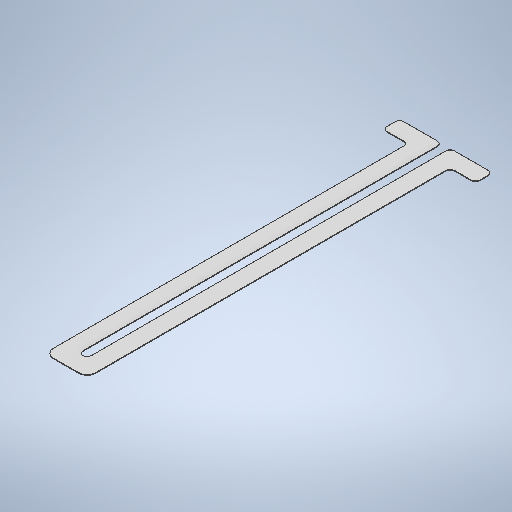
# Autodesk Inventor part: Lungo
Saved by Autodesk Inventor 2025.4 (Build 294407000, 407)
## iProperties
Created: 2026-04-15
Part Number: Lungo
Material: Generic
Document SubType Name: Modeling
Designer: gdira
Density: 1 g/cm^3
Appearance: Default
Author: gdira
Autodesk Inventor part; units mm, degrees
ref_plane "YZ Plane" through (0, 0, 0) normal (1, 0, 0) x (0, 1, 0)
ref_plane "XZ Plane" through (0, 0, 0) normal (0, 1, 0) x (-1, 0, 0)
ref_plane "XY Plane" through (0, 0, 0) normal (0, 0, 1) x (1, 0, 0)
sketch "Sketch1" plane through (0, 0, 0) normal (0, 1, 0) x (-1, 0, 0)
  line L0 (0.1981, -3.9947) -> (-1.7926, -3.9947)
  line L1 (-5.7926, -3.9915) -> (-13.7926, -3.9915)
  line L2 (0.1981, -3.9947) -> (6.2092, -3.9837)
  line L3 (-4.7926, 81.0108) -> (-4.7926, -2.9915)
  line L4 (-2.7926, -2.9947) -> (-2.7926, 81.0108)
  line L5 (-3.7926, 82.0108) -> (-3.7926, 82.0108)
  line L6 (-8.7926, 84.0108) -> (-8.7926, 4.0085)
  line L7 (-6.7926, 86.0108) -> (-0.7926, 86.0108)
  line L8 (1.2074, 84.0108) -> (1.2074, 4.0363)
  arc A0 (-6.7926, 86.0108) -> (-8.7926, 84.0108) centre (-6.7926, 84.0108) ccw
  arc A1 (1.2074, 84.0108) -> (-0.7926, 86.0108) centre (-0.7926, 84.0108) ccw
  line L9 (7.2074, -2.9837) -> (7.2074, -0.9819)
  line L10 (6.2074, 0.0181) -> (2.2074, 0.0181)
  line L11 (1.2074, 1.0181) -> (1.2074, 7.5905)
  line L12 (-14.7926, -2.9915) -> (-14.7926, -0.9915)
  line L13 (-13.7926, 0.0085) -> (-9.7926, 0.0085)
  line L14 (-8.7926, 1.0085) -> (-8.7926, 4.0085)
  arc A2 (-9.7926, 0.0085) -> (-8.7926, 1.0085) centre (-9.7926, 1.0085) ccw
  arc A3 (-13.7926, 0.0085) -> (-14.7926, -0.9915) centre (-13.7926, -0.9915) ccw
  arc A4 (-14.7926, -2.9915) -> (-13.7926, -3.9915) centre (-13.7926, -2.9915) ccw
  arc A5 (-5.7926, -3.9915) -> (-4.7926, -2.9915) centre (-5.7926, -2.9915) ccw
  arc A6 (-2.7926, -2.9947) -> (-1.7926, -3.9947) centre (-1.7926, -2.9947) ccw
  arc A7 (6.2092, -3.9837) -> (7.2074, -2.9837) centre (6.2074, -2.9837) ccw
  arc A8 (7.2074, -0.9819) -> (6.2074, 0.0181) centre (6.2074, -0.9819) ccw
  arc A9 (1.2074, 1.0181) -> (2.2074, 0.0181) centre (2.2074, 1.0181) ccw
  arc A10 (-3.7926, 82.0108) -> (-4.7926, 81.0108) centre (-3.7926, 81.0108) ccw
  arc A11 (-2.7926, 81.0108) -> (-3.7926, 82.0108) centre (-3.7926, 81.0108) ccw
  point P0 (0, 0)
  point P1 (0.8878, 16.4413)
  point P2 (-2.7926, -3.9947)
  point P3 (3.2037, -3.9892)
  point P4 (-14.7926, -3.9915)
  point P5 (7.2074, -3.9819)
  point P6 (-3.7926, 82.0108)
  point P7 (-3.7926, 86.0108)
  point P8 (7.2074, 0.0181)
  point P9 (-14.7926, 0.0085)
  point P10 (1.2074, 4.0363)
  dimension "d0" = 10
  dimension "d1" = 4
  dimension "d2" = 4
  dimension "d3" = 2
  dimension "d4" = 4
  dimension "d5" = 90
  dimension "d6" = 2
  dimension "d7" = 4
  dimension "d8" = 4
  dimension "d9" = 1
  dimension "d10" = 1
  constraints: 30 end point, 24 point on circle, 24 tangent, 12 centre point, 11 point on line, 9 equal radius, 5 perpendicular, 3 midpoint, 2 horizontal, 2 vertical, 1 collinear, 1 parallel
  measures "d0" distance of point (7.207, -3.982) point (-2.793, -3.995)
  measures "d1" distance between parallel lines of L4 L8
  measures "d2" distance between parallel lines of L6 L3
  measures "d3" distance between parallel lines of L3 L4
  measures "d4" distance of point (-3.793, 86.011) point (-3.793, 82.011)
  measures "d5" distance from line of point (3.204, -3.989) L7
  measures "d6" radius of A0
  measures "d7" distance of point (7.207, -3.982) point (7.207, 0.018)
  measures "d8" distance of point (-14.793, -3.992) point (-14.793, 0.008)
  measures "d9" radius of A2
  measures "d10" radius of A10
extrude "Extrusion1" add sketch "Sketch1" along normal blind 0.15
body "Solid1"
